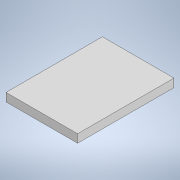
# Autodesk Inventor part: placa centro
Saved by Autodesk Inventor 2021.2 (Build 252289000, 289)
## iProperties
Created: 2021-04-11
Part Number: placa centro
Material: Genérico
Document SubType Name: Modeling
Designer: equip
Density: 1 g/cm^3
Appearance: Valor por defecto
Mass: 341.25 g
Surface Area: 546.5 cm^2
Volume: 341.25 cm^3
Author: equip
Autodesk Inventor part; units mm, degrees
ref_plane "YZ Plane" through (0, 0, 0) normal (1, 0, 0) x (0, 1, 0)
ref_plane "XZ Plane" through (0, 0, 0) normal (0, 1, 0) x (-1, 0, 0)
ref_plane "XY Plane" through (0, 0, 0) normal (0, 0, 1) x (1, 0, 0)
sketch "Boceto1" plane through (0, 0, 0) normal (0, 1, 0) x (-1, 0, 0)
  line L0 (70.1489, 81.5719) -> (-59.8511, 81.5719)
  line L1 (-59.8511, 81.5719) -> (-59.8511, -93.4281)
  line L2 (-59.8511, -93.4281) -> (70.1489, -93.4281)
  line L3 (70.1489, -93.4281) -> (70.1489, 81.5719)
  point P0 (0, 0)
  dimension "d0" = 130
  dimension "d1" = 175
  constraints: 8 end point, 2 parallel, 1 horizontal, 1 perpendicular
  measures "d0" distance of L2.end L1.end
  measures "d1" distance of L1.end L0.end
extrude "Extrusión1" add sketch "Boceto1" along normal blind 15
